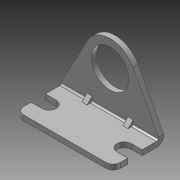
# Autodesk Inventor part: Rebuild Shooter NCDME075-0600 Cylinder Mounting Bracket
Saved by Autodesk Inventor 2014 SP1 (Build 180222100, 222)
## iProperties
Category: PARTsolutions
Company: BIMBA
Created: 2013-01-26
Part Number: Rebuild Shooter NCDME075-0600 Cylinder Mounting Bracket
Material: Steel
Catalog Web Link: www.cadenas.de
Description: Mounting Brackets for Original Line Cylinders-
Vendor: BIMBA
Document SubType Name: Modeling
Designer: actoennies
Manufacturer: BIMBA
Density: 7.85 g/cm^3
Mass: 25.0496 g
Surface Area: 33.3295 cm^2
Volume: 3.19103 cm^3
Appearance: Steel
PSOL_IDENT_0: {\\10.0.0.242\data_v9\23d-libs\bimba\bimba\bimba_imperial\bimba_full_line\original_line_cylinders\ac
PSOL_IDENT_1: cessories\mounting_bracket.prj},191 {VTYP=3D},{NB=D-770},{LINA=D-770},{NN=Mounting Brackets for Orig
PSOL_IDENT_2: inal Line Cylinders},{DATE=26.09.2012 12:25:43},{GEOMDATE=27.08.2012 00:00:00},{VERSION=},{LINEID=40
PSOL_IDENT_3: },{LINESUBID=-1},{WBVAR=}  {NB=D-770},{LINA=D-770},{KT=DUMMY},{PN=D-770},{PSPN=0.44 (D-770)},{PN1=D-
PSOL_IDENT_4: 770},{MAT=Zinc-Plated Carbon Steel},{A=0.83},{A1=0.82900},{B=1.38},{B1=1.37500},{C=0.69},{C1=0.69000
PSOL_IDENT_5: },{D=0.44},{D1=0.44050},{E=0.19},{E1=0.19200},{F=0.38},{F1=0.38000},{G=0.56},{G1=0.56170},{H=0.09},{
PSOL_IDENT_6: H1=0.08970},{I=0.38},{I1=0.37500},{J=1.00},{J1=1.00000},{K=0.13},{K1=0.12500},{L=0.13},{L1=0.12500},
PSOL_IDENT_7: {M=0.03100},{N=0.00000},{SHP=3},{ASSCFGPRA=mounting_bracket3},{COLOR=0.75,0.75,0.75,0.00}
CNS_NB: D-770
CNS_NBSYN: $PN1.
CNS_LINA: D-770
CNS_PN: D-770
CNS_PSPN: ø.44 (D-770)
CNS_PN1: D-770
CNS_MAT: Zinc-Plated Carbon Steel
CNS_A: 0.83
CNS_A1: 0.82900
CNS_B: 1.38
CNS_B1: 1.37500
CNS_C: 0.69
CNS_C1: 0.69000
CNS_D: 0.44
CNS_D1: 0.44050
CNS_E: 0.19
CNS_E1: 0.19200
CNS_F: 0.38
CNS_F1: 0.38000
CNS_G: 0.56
CNS_G1: 0.56170
CNS_H: 0.09
CNS_H1: 0.08970
CNS_I: 0.38
CNS_I1: 0.37500
CNS_J: 1.00
CNS_J1: 1.00000
CNS_K: 0.13
CNS_K1: 0.12500
CNS_L: 0.13
CNS_L1: 0.12500
CNS_M: 0.03100
CNS_N: 0.00000
CNS_SHP: 3
CNS_ASSCFGPRA: mounting_bracket3
CNS_COLOR: 0.75,0.75,0.75,0.00
SUPPLIER: BIMBA
ARTICLENO: D-770
BOMINFO: D-770
CREATOR: CADENAS GmbH
Title: D-770
Author: Cadenas PARTsolutions
Autodesk Inventor part; units mm, degrees
sketch "Sketch_1" plane through (0, 0, 0) normal (1, 0, 0) x (0, 1, 0)
  line L0 (0, 22.225) -> (0, 3.0658)
  arc A0 (0, 3.0658) -> (3.0658, 0) centre (3.0658, 3.0658) ccw
  line L1 (3.0658, 0) -> (31.6408, 0)
  line L2 (31.6408, 0) -> (31.6408, 2.2784)
  line L3 (31.6408, 2.2784) -> (3.0658, 2.2784)
  arc A1 (2.2784, 3.0658) -> (3.0658, 2.2784) centre (3.0658, 3.0658) ccw
  line L4 (2.2784, 3.0658) -> (2.2784, 22.225)
  line L5 (2.2784, 22.225) -> (0, 22.225)
  dimension "d36" = 28.575
  dimension "d37" = 3.0658
  dimension "d38" = 0.7874
  dimension "d40" = 2.2784
  dimension "d43" = 22.225
  constraints: 12 end point, 4 point on circle, 4 tangent, 3 vertical, 2 centre point, 2 equal length, 2 horizontal, 1 other
  measures "d36" distance of L1.start L1.end
  measures "d37" radius of A0
  measures "d38" radius of A1
  measures "d40" distance of L4.end L0.start
  measures "d43" distance from line of L5 L1.start
extrude "Extrusion1" add sketch "Sketch_1" along normal blind 42.545
sketch "Sketch_2" plane through (0, 0, 0) normal (0, 0, 1) x (1, 0, 0)
  line L0 (-3.175, -2.1057) -> (45.72, -2.1057)
  line L1 (45.72, -2.1057) -> (45.72, 33.6906)
  line L2 (45.72, 33.6906) -> (-3.175, 33.6906)
  line L3 (-3.175, 33.6906) -> (-3.175, -2.1057)
  line L4 (-1.905, 0) -> (44.45, 0)
  line L5 (44.45, 0) -> (31.3469, 24.4492)
  arc A0 (31.3469, 24.4492) -> (11.1981, 24.4492) centre (21.2725, 19.05) ccw
  line L6 (11.1981, 24.4492) -> (-1.905, 0)
  line L7 (0, 0) -> (0, 3.0658) construction
  line L8 (0, 3.0658) -> (42.545, 3.0658) construction
  line L9 (42.545, 0) -> (42.545, 3.0658) construction
  line L10 (0, 0) -> (42.545, 0) construction
  line L11 (21.2725, 19.05) -> (21.2725, 0) construction
  line L12 (21.2725, 0) -> (21.2725, -2.1057) construction
  dimension "d23" = 46.355
  dimension "d24" = 11.43
  dimension "d25" = 19.05
  dimension "d26" = 35.7962
  dimension "d27" = 48.895
  dimension "d30" = 2.1057
  constraints: 18 end point, 3 vertical, 2 horizontal, 2 midpoint, 2 perpendicular, 2 point on circle, 2 tangent, 1 centre point, 1 equal length, 1 point on line
  measures "d23" distance of L4.start L4.end
  measures "d24" radius of A0
  measures "d25" distance from line of L4 L11.start
  measures "d26" distance of L0.end L1.end
  measures "d27" distance of L1.end L2.end
  measures "d30" distance of L11.end L12.end
extrude "Extrusion2" cut sketch "Sketch_2" along normal blind 3.4176
sketch "Sketch3" plane through (42.545, 3.0658, 0) normal (0, 0, -1) x (-1, 0, 0)
  arc A0 (31.3469, 21.3834) -> (11.1981, 21.3834) centre (21.2725, 15.9842) ccw projected
  constraints: 1 coincident
hole "Drilling 1" at (21.2725, 19.05, 0) direction (0, 0, 1) diameter 16.51 depth 3.4176
sketch "Sketch_8" plane through (0, 0, 0) normal (0, 1, 0) x (-1, 0, 0)
  line L0 (3.4925, 15.7658) -> (-4.7625, 15.7658)
  arc A0 (-4.7625, 15.7658) -> (-4.7625, 9.4158) centre (-4.7625, 12.5908) ccw
  line L1 (-4.7625, 9.4158) -> (3.4925, 9.4158)
  line L2 (3.4925, 9.4158) -> (3.4925, 15.7658)
  line L3 (0, 3.0658) -> (-42.545, 3.0658) projected
  dimension "d31" = 3.4925
  dimension "d32" = 8.255
  dimension "d33" = 3.175
  dimension "d34" = 6.35
  dimension "d35" = 6.35
  constraints: 6 end point, 2 point on circle, 2 tangent, 1 centre point, 1 parallel, 1 vertical
  measures "d31" distance from line of L2 L3.start
  measures "d32" distance of L1.start L1.end
  measures "d33" radius of A0
  measures "d34" distance of L1.end L0.start
  measures "d35" distance from line of L1 L3.start
extrude "Extrusion5" cut sketch "Sketch_8" along normal blind 3.4176
sketch "Sketch_10" plane through (11.1125, 0, 0) normal (1, 0, 0) x (0, 0, -1)
  arc A0 (-4.5568, 1.8456) -> (-1.8456, 4.5568) centre (-3.0658, 3.0658) ccw
  line L0 (-1.8456, 4.5568) -> (-2.2784, 4.5568)
  line L1 (-2.2784, 4.5568) -> (-4.5568, 2.2784)
  line L2 (-4.5568, 2.2784) -> (-4.5568, 1.8456)
  constraints: 6 end point, 2 point on circle, 1 centre point
extrude "Extrusion7" add sketch "Sketch_10" along normal blind 2.2784
ref_plane "h1_XY" through (17.4625, 0, 17.526) normal (1, 0, 0) x (0, 0, -1)
ref_plane "h1_YZ" through (17.4625, 0, 17.526) normal (0, 0, -1) x (0, 1, 0)
ref_plane "h1_ZX" through (17.4625, 0, 17.526) normal (0, 1, 0) x (1, 0, 0)
ref_plane "d1_XY" through (17.4625, 8.6728, 0) normal (1, 0, 0) x (0, 0, -1)
ref_plane "d1_YZ" through (17.4625, 8.6728, 0) normal (0, 0, -1) x (0, 1, 0)
ref_plane "d1_ZX" through (17.4625, 8.6728, 0) normal (0, 1, 0) x (1, 0, 0)
ref_plane "h2_XY" through (17.4625, 2.2784, 17.526) normal (1, 0, 0) x (0, 0, -1)
ref_plane "h2_YZ" through (17.4625, 2.2784, 17.526) normal (0, 0, -1) x (0, 1, 0)
ref_plane "h2_ZX" through (17.4625, 2.2784, 17.526) normal (0, 1, 0) x (1, 0, 0)
ref_plane "d2_XY" through (17.4625, 19.8615, 0) normal (1, 0, 0) x (0, 0, -1)
ref_plane "d2_YZ" through (17.4625, 19.8615, 0) normal (0, 0, -1) x (0, 1, 0)
ref_plane "d2_ZX" through (17.4625, 19.8615, 0) normal (0, 1, 0) x (1, 0, 0)
ref_plane "h3_XY" through (17.4625, 14.2672, 2.2784) normal (1, 0, 0) x (0, 0, -1)
ref_plane "h3_YZ" through (17.4625, 14.2672, 2.2784) normal (0, 0, -1) x (0, 1, 0)
ref_plane "h3_ZX" through (17.4625, 14.2672, 2.2784) normal (0, 1, 0) x (1, 0, 0)
ref_plane "h4_XY" through (17.4625, 21.0566, 2.2784) normal (1, 0, 0) x (0, 0, -1)
ref_plane "h4_YZ" through (17.4625, 21.0566, 2.2784) normal (0, 0, -1) x (0, 1, 0)
ref_plane "h4_ZX" through (17.4625, 21.0566, 2.2784) normal (0, 1, 0) x (1, 0, 0)
ref_plane "h5_XY" through (34.925, 3.175, 0) normal (1, 0, 0) x (0, 0, -1)
ref_plane "h5_YZ" through (34.925, 3.175, 0) normal (0, 0, -1) x (0, 1, 0)
ref_plane "h5_ZX" through (34.925, 3.175, 0) normal (0, 1, 0) x (1, 0, 0)
ref_plane "h6_XY" through (34.925, 0, 0) normal (1, 0, 0) x (0, 0, -1)
ref_plane "h6_YZ" through (34.925, 0, 0) normal (0, 0, -1) x (0, 1, 0)
ref_plane "h6_ZX" through (34.925, 0, 0) normal (0, 1, 0) x (1, 0, 0)
ref_plane "l1_XY" through (0, 0, 0) normal (0, 1, 0) x (1, 0, 0)
ref_plane "l1_YZ" through (0, 0, 0) normal (1, 0, 0) x (0, 0, -1)
ref_plane "l1_ZX" through (0, 0, 0) normal (0, 0, -1) x (0, 1, 0)
ref_plane "l2_XY" through (34.925, 0, 0) normal (0, 1, 0) x (1, 0, 0)
ref_plane "l2_YZ" through (34.925, 0, 0) normal (1, 0, 0) x (0, 0, -1)
ref_plane "l2_ZX" through (34.925, 0, 0) normal (0, 0, -1) x (0, 1, 0)
ref_plane "l3_XY" through (0, 0, 17.526) normal (0, 1, 0) x (1, 0, 0)
ref_plane "l3_YZ" through (0, 0, 17.526) normal (1, 0, 0) x (0, 0, -1)
ref_plane "l3_ZX" through (0, 0, 17.526) normal (0, 0, -1) x (0, 1, 0)
ref_plane "l4_XY" through (0, 0, 9.652) normal (0, 1, 0) x (1, 0, 0)
ref_plane "l4_YZ" through (0, 0, 9.652) normal (1, 0, 0) x (0, 0, -1)
ref_plane "l4_ZX" through (0, 0, 9.652) normal (0, 0, -1) x (0, 1, 0)
ref_plane "l5_XY" through (4.7625, 0, 9.652) normal (0, 1, 0) x (1, 0, 0)
ref_plane "l5_YZ" through (4.7625, 0, 9.652) normal (1, 0, 0) x (0, 0, -1)
ref_plane "l5_ZX" through (4.7625, 0, 9.652) normal (0, 0, -1) x (0, 1, 0)
ref_plane "l6_XY" through (30.1625, 0, 9.652) normal (0, 1, 0) x (1, 0, 0)
ref_plane "l6_YZ" through (30.1625, 0, 9.652) normal (1, 0, 0) x (0, 0, -1)
ref_plane "l6_ZX" through (30.1625, 0, 9.652) normal (0, 0, -1) x (0, 1, 0)
ref_plane "l7_XY" through (30.1625, 0, 12.0904) normal (0, 1, 0) x (1, 0, 0)
ref_plane "l7_YZ" through (30.1625, 0, 12.0904) normal (1, 0, 0) x (0, 0, -1)
ref_plane "l7_ZX" through (30.1625, 0, 12.0904) normal (0, 0, -1) x (0, 1, 0)
ref_plane "l8_XY" through (30.1625, 0, 7.2136) normal (0, 1, 0) x (1, 0, 0)
ref_plane "l8_YZ" through (30.1625, 0, 7.2136) normal (1, 0, 0) x (0, 0, -1)
ref_plane "l8_ZX" through (30.1625, 0, 7.2136) normal (0, 0, -1) x (0, 1, 0)
ref_plane "mounting_bracket_XY" through (17.4625, 14.2672, 2.2784) normal (0, 0, 1) x (1, 0, 0)
ref_plane "mounting_bracket_YZ" through (17.4625, 14.2672, 2.2784) normal (1, 0, 0) x (0, 1, 0)
ref_plane "mounting_bracket_ZX" through (17.4625, 14.2672, 2.2784) normal (0, 1, 0) x (0, 0, 1)
ref_plane "mounting_bracket_1_XY" through (17.4625, 14.2672, 0) normal (0, 0, 1) x (1, 0, 0)
ref_plane "mounting_bracket_1_YZ" through (17.4625, 14.2672, 0) normal (1, 0, 0) x (0, 1, 0)
ref_plane "mounting_bracket_1_ZX" through (17.4625, 14.2672, 0) normal (0, 1, 0) x (0, 0, 1)
fillet "Fillet1" radius 3.175 1 edges at (0, 1.1392, 22.225)
ref_plane "Work Plane56" through (21.2725, 0, 0) normal (1, 0, 0) x (0, 0, -1)
mirror "Mirror2" about plane through (21.2725, 0, 0) normal (1, 0, 0) of "Extrusion5", "Fillet1", "Extrusion7"
equation "\"d33\" = 0.5 * d34"
body "Solid1"
